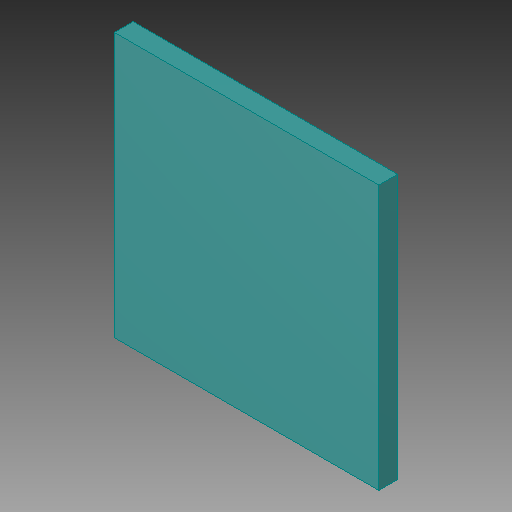
# Autodesk Inventor part: E5-13
Saved by Autodesk Inventor 2017 (Build 210142000, 142)
## iProperties
Created: 2019-06-13
Part Number: E5-13
Material: Generic
Document SubType Name: Modeling
Designer: Marc
Density: 1 g/cm^3
Appearance: E5-13, E5-13
Author: Marc
Autodesk Inventor part; units mm, degrees
ref_plane "YZ Plane" through (0, 0, 0) normal (1, 0, 0) x (0, 1, 0)
ref_plane "XZ Plane" through (0, 0, 0) normal (0, 1, 0) x (-1, 0, 0)
ref_plane "XY Plane" through (0, 0, 0) normal (0, 0, 1) x (1, 0, 0)
sketch "E5-13, E5-13_5" plane through (0, 0, 0) normal (0, 0, 1) x (1, 0, 0)
  line L0 (-7.0612, 7.0612) -> (7.0612, 7.0612)
  line L1 (7.0612, 7.0612) -> (7.0612, -7.0612)
  line L2 (7.0612, -7.0612) -> (-7.0612, -7.0612)
  line L3 (-7.0612, -7.0612) -> (-7.0612, 7.0612)
  constraints: 8 end point
extrude "Extrusion1" add sketch "E5-13, E5-13_5" along normal blind 1
body "Solid1"
